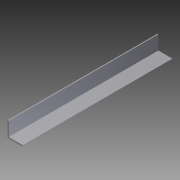
# Autodesk Inventor part: 8 ball  frame corner L
Saved by Autodesk Inventor 2012 (Build 160160000, 160)
## iProperties
Created: 2013-10-18
Part Number: 8 ball  frame corner L
Material: Default
Document SubType Name: Modeling
Designer: Bryce
Density: 1 g/cm^3
Author: Bryce
Autodesk Inventor part; units mm, degrees
ref_plane "YZ Plane" through (0, 0, 0) normal (1, 0, 0) x (0, 1, 0)
ref_plane "XZ Plane" through (0, 0, 0) normal (0, 1, 0) x (-1, 0, 0)
ref_plane "XY Plane" through (0, 0, 0) normal (0, 0, 1) x (1, 0, 0)
sketch "Sketch1" plane through (0, 0, 0) normal (0, 0, 1) x (1, 0, 0)
  line L0 (0, 0) -> (25.3902, 0)
  line L1 (25.3902, 0) -> (25.3902, 1.5875)
  line L2 (1.5875, 25.4) -> (0, 25.4)
  line L3 (0, 25.4) -> (0, 0)
  line L4 (1.5875, 25.4) -> (1.5875, 1.5875)
  line L5 (1.5875, 1.5875) -> (25.3902, 1.5875)
  dimension "d0" = 25.4
  dimension "d1" = 25.3902
  dimension "d2" = 1.5875
  dimension "d3" = 1.5875
  constraints: 12 end point, 2 parallel, 1 horizontal, 1 perpendicular
  measures "d0" distance of L2.end L0.start
  measures "d1" distance of L0.start L0.end
  measures "d2" distance between parallel lines of L0 L5
  measures "d3" distance between parallel lines of L3 L4
extrude "Extrusion1" add sketch "Sketch1" along normal blind 254
equation "\"d2\" = d3"
body "Solid1"
